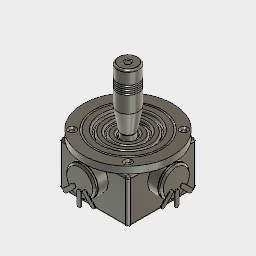
3102 Mini Joystick (Autodesk Fusion 360 design; units mm, degrees)
Autodesk Fusion 360 part; units mm, degrees
note: some values were not read from the file. Chosen so that the rebuilt part matches the saved one: which face or edge a step refers to. Set by a fixed rule: which sketch regions a step uses.
sketch "base" plane through (0, 0, 0) normal (0, 0, 1) x (1, 0, 0)
  circle A0 centre (0, 0) radius 19.8
  line L0 (16.25, -16.25) -> (-16.25, -16.25) construction
  line L1 (-16.25, -16.25) -> (-16.25, 16.25) construction
  line L2 (-16.25, 16.25) -> (16.25, 16.25) construction
  line L3 (16.25, 16.25) -> (16.25, -16.25) construction
  line L4 (16.25, -16.25) -> (-16.25, 16.25) construction
  line L5 (-16.25, -16.25) -> (16.25, 16.25) construction
  circle A1 centre (-16.25, 16.25) radius 1.25
  circle A2 centre (16.25, 16.25) radius 1.25
  circle A3 centre (16.25, -16.25) radius 1.25
  circle A4 centre (-16.25, -16.25) radius 1.25
  circle A5 centre (0, 0) radius 26
  dimension "d1" = 39.6
  dimension "d7" = 32.5
  dimension "d8" = 32.5
  dimension "d9" = 2.5
  dimension "d10" = 2.5
  dimension "d11" = 2.5
  dimension "d12" = 2.5
  dimension "d13" = 52
  measures "d1" diameter of A0
  measures "d7" distance of L1.end L2.end
  measures "d8" distance of L0.end L1.end
  measures "d9" diameter of A1
  measures "d10" diameter of A2
  measures "d11" diameter of A3
  measures "d12" diameter of A4
  measures "d13" diameter of A5
extrude "Extrude1" add sketch "base" along normal blind 4 makes body 1
sketch "stick" plane through (0, 0, 4) normal (0, 0, 1) x (-1, 0, 0)
  circle A0 centre (0, 0) radius 19.8
  circle A1 centre (0, 0) radius 4
  circle A2 centre (16.25, 16.25) radius 1.25
  circle A3 centre (16.25, -16.25) radius 1.25
  circle A4 centre (-16.25, -16.25) radius 1.25
  circle A5 centre (-16.25, 16.25) radius 1.25
  circle A6 centre (0, 0) radius 26
  dimension "d4" = 8
  measures "d4" diameter of A1
extrude "Extrude2" add sketch "stick" along normal blind 12 draft 10 separate body contours A1 makes body 2
sketch "rod" plane through (0, 0, 16) normal (0, 0, 1) x (-1, 0, 0)
  circle A0 centre (0, 0) radius 6.1159
extrude "Extrude3" add sketch "rod" along normal blind 22 bodies 2
sketch "pad (1)" plane through (0, 0, 0) normal (0, 0, 1) x (1, 0, 0)
  circle A0 centre (0, 0) radius 26
  circle A1 centre (0, 0) radius 4
  circle A2 centre (0, 0) radius 26
  circle A3 centre (0, 0) radius 19.8
  circle A4 centre (0, 0) radius 16
  circle A5 centre (0, 0) radius 12
  circle A6 centre (0, 0) radius 8
  dimension "d16" = 10
  dimension "d17" = 14
  dimension "d18" = 18
  dimension "d50" = 8
  dimension "d104" = 39.6
  measures "d50" diameter of A1
  measures "d104" diameter of A3
extrude "pad" add sketch "pad (1)" along normal blind 3 separate body contours A3 | A4 | A5 | A6 makes body 3
pipe "Pipe6" cut diameter 2 path "pad (1)" along A6 bodies 3
pipe "Pipe7" cut diameter 2 path "pad (1)" along A5 bodies 3
pipe "Pipe8" cut diameter 2 path "pad (1)" along A4 bodies 3
move_body "Move1" bodies 3 to x (-1, 0, 0) y (0, 1, 0) z (0, 0, -1) at (0, 0, 3)
ref_plane "WorkPlane1" through (0, 0, 26) normal (0, 0, 1) x (-1, 0, 0)
sketch "rings" plane through (0, 0, 26) normal (0, 0, 1) x (1, 0, 0)
  circle A0 centre (0, 0) radius 6.1159
pipe "Pipe5" cut diameter 1 path "rings" along A0 bodies 2
pattern_linear "R-Pattern1" count 3 spacing 2 along (0, 0, 1) of 1 faces at (-6.0834, 0.3036, 26.4994) on bodies 2
fillet "Fillet1" radius 1 1 edges at (5.702, 2.2116, 38) on bodies 2
extrude "Extrude5" add sketch "pad (1)" along normal blind 4 draft -10 separate body contours A1 makes body 4
fillet "Fillet2" radius 1 1 edges at (-3.0717, 1.1914, 4) on bodies 4
chamfer "Chamfer1" distance 1 angle 45 4 edges at (-17.4154, 16.702, 4) (15.0846, 16.702, 4) (-17.4154, -15.798, 4) (15.0846, -15.798, 4) on bodies 1
sketch "Sketch6" plane through (0, 0, 0) normal (0, 0, 1) x (1, 0, 0)
  line L0 (20, -20) -> (-20, -20)
  line L1 (-20, -20) -> (-20, 20)
  line L2 (-20, 20) -> (20, 20)
  line L3 (20, 20) -> (20, -20)
  line L4 (20, -20) -> (-20, 20) construction
  line L5 (-20, -20) -> (20, 20) construction
  dimension "d74" = 40
  dimension "d75" = 40
  measures "d74" distance of L1.end L2.end
  measures "d75" distance of L0.end L1.end
extrude "Extrude15" add sketch "Sketch6" against normal blind 26 separate body makes body 5
fillet "Fillet4" radius 1.5 12 edges at (20, 20, -13) (-20, 0, 0) (0, -20, -26) (20, 0, -26) (20, 0, 0) (0, 20, -26) (-20, 20, -13) (0, 20, 0) (-20, -20, -13) (0, -20, 0) (20, -20, -13) (-20, 0, -26) on bodies 5
sketch "pot a" plane through (20, 0, 0) normal (1, 0, 0) x (0, 1, 0)
  line L0 (-18.5, -1.5) -> (-18.5, -24.5)
  line L1 (-18.5, -24.5) -> (18.5, -24.5)
  line L2 (18.5, -24.5) -> (18.5, -1.5)
  line L3 (18.5, -1.5) -> (-18.5, -1.5)
  line L4 (0, -24.5) -> (0, -1.5) construction
  circle A0 centre (0, -8.5) radius 8.5
  dimension "d81" = 17
  dimension "d89" = 16
  measures "d81" diameter of A0
  measures "d89" distance of L1 A0.centre
extrude "Extrude16" add sketch "pot a" along normal blind 6 separate body contours L3 A0 | L3 A0 makes body 6
sketch "pot b" plane through (0, -20, 0) normal (0, -1, 0) x (1, 0, 0)
  line L0 (18.5, -1.5) -> (-18.5, -1.5)
  line L1 (-18.5, -1.5) -> (-18.5, -24.5)
  line L2 (-18.5, -24.5) -> (18.5, -24.5)
  line L3 (18.5, -24.5) -> (18.5, -1.5)
  line L4 (0, -1.5) -> (0, -24.5) construction
  circle A0 centre (0, -8.5) radius 8.5
  dimension "d85" = 17
  dimension "d86" = 16
  measures "d85" diameter of A0
  measures "d86" distance of L2 A0.centre
extrude "Extrude17" add sketch "pot b" along normal blind 6 separate body contours L0 A0 | L0 A0 makes body 7
fillet "Fillet5" radius 1 1 edges at (3.7293, 1.4465, 3) on bodies 3
sketch "bottom hole" plane through (0, 0, -26) normal (0, 0, -1) x (1, 0, 0)
  line L0 (18.5, -18.5) -> (18.5, 18.5)
  line L1 (18.5, 18.5) -> (-18.5, 18.5)
  line L2 (-18.5, 18.5) -> (-18.5, -18.5)
  line L3 (-18.5, -18.5) -> (18.5, -18.5)
  circle A0 centre (0, 0) radius 9.5
  dimension "d106" = 19
  measures "d106" diameter of A0
extrude "Extrude18" cut sketch "bottom hole" against normal blind 2 contours A0 bodies 5
sketch "top dimple" plane through (0, 0, 38) normal (0, 0, 1) x (-1, 0, 0)
  circle A0 centre (0, 0) radius 5.1159
  circle A1 centre (0, 0) radius 1.5
  dimension "d109" = 3
  measures "d109" diameter of A1
extrude "Extrude19" cut sketch "top dimple" against normal blind 0.5 contours A1 bodies 2
fillet "Fillet6" radius 0.5 1 edges at (1.3985, -0.5424, 38) on bodies 2
extrude "Extrude20" add sketch "pot b" along normal blind 2 from surface at 6 separate body contours L0 A0 | L0 A0 makes body 8
extrude "Extrude21" add sketch "pot a" along normal blind 2 from surface at 6 separate body contours L3 A0 | L3 A0 makes body 9
chamfer "Chamfer3" distance 1 angle 45 2 edges at (-7.9248, -28, -11.5737) (28, -7.9248, -11.5737) on bodies 8 9
chamfer "Chamfer4" distance 0.25 angle 45 2 edges at (26, -7.9248, -11.5737) (-7.9248, -26, -11.5737) on bodies 6 7
sketch "Sketch12" plane through (0, -28, 0) normal (0, -1, 0) x (1, 0, 0)
  circle A0 centre (0, -8.5) radius 7.5
  circle A1 centre (0, -8.5) radius 2
  line L0 (-1.2, -13.2) -> (-1.2, -19.8)
  arc A2 (-1.2, -19.8) -> (1.2, -19.8) centre (0, -19.8) ccw
  line L1 (1.2, -19.8) -> (1.2, -13.2)
  arc A3 (1.2, -13.2) -> (-1.2, -13.2) centre (0, -13.2) ccw
  line L2 (0, -12) -> (0, -21) construction
  line L3 (2.4749, -12.6719) -> (7.1418, -17.3388)
  arc A4 (7.1418, -17.3388) -> (8.8388, -15.6418) centre (7.9903, -16.4903) ccw
  arc A5 (4.1719, -10.9749) -> (2.4749, -12.6719) centre (3.3234, -11.8234) ccw
  line L4 (8.8388, -15.6418) -> (4.1719, -10.9749)
  line L5 (-8.8388, -15.6418) -> (-4.1719, -10.9749)
  arc A6 (-2.4749, -12.6719) -> (-4.1719, -10.9749) centre (-3.3234, -11.8234) ccw
  line L6 (-2.4749, -12.6719) -> (-7.1418, -17.3388)
  arc A7 (-8.8388, -15.6418) -> (-7.1418, -17.3388) centre (-7.9903, -16.4903) ccw
  dimension "d121" = 4
  dimension "d122" = 2.4
  dimension "d124" = 45
  measures "d121" diameter of A1
  measures "d122" diameter of A2
extrude "Extrude22" add sketch "Sketch12" along normal blind 0.5 separate body contours A0 L5 A6 L6 | A0 L5 L6 A7 | A0 L3 A4 L4 | A0 L3 A5 L4 | A0 L0 L1 A3 | A0 L0 A2 L1 makes body 10 at (-4.5962, -28, -13.6619) makes body 11 at (0.4, -28, -15.4) makes body 12 at (4.5962, -28.5, -13.6619)
sketch "Sketch13" plane through (28, 0, 0) normal (1, 0, 0) x (0, 1, 0)
  circle A0 centre (0, -8.5) radius 7.5
  circle A1 centre (0, -8.5) radius 2
  line L0 (-1.2, -13.2) -> (-1.2, -19.8)
  arc A2 (-1.2, -19.8) -> (1.2, -19.8) centre (0, -19.8) ccw
  line L1 (1.2, -19.8) -> (1.2, -13.2)
  arc A3 (1.2, -13.2) -> (-1.2, -13.2) centre (0, -13.2) ccw
  line L2 (0, -12) -> (0, -21) construction
  line L3 (2.4749, -12.6719) -> (7.1418, -17.3388)
  arc A4 (7.1418, -17.3388) -> (8.8388, -15.6418) centre (7.9903, -16.4903) ccw
  line L4 (8.8388, -15.6418) -> (4.1719, -10.9749)
  arc A5 (4.1719, -10.9749) -> (2.4749, -12.6719) centre (3.3234, -11.8234) ccw
  line L5 (-8.8388, -15.6418) -> (-4.1719, -10.9749)
  arc A6 (-2.4749, -12.6719) -> (-4.1719, -10.9749) centre (-3.3234, -11.8234) ccw
  arc A7 (-8.8388, -15.6418) -> (-7.1418, -17.3388) centre (-7.9903, -16.4903) ccw
  line L6 (-2.4749, -12.6719) -> (-7.1418, -17.3388)
  dimension "d127" = 4
  dimension "d128" = 2.4
  dimension "d130" = 45
  measures "d127" diameter of A1
  measures "d128" diameter of A2
extrude "Extrude23" add sketch "Sketch13" along normal blind 0.5 separate body contours A0 L5 A6 L6 | A0 L5 A7 L6 | A0 L3 A4 L4 | A0 L3 L4 A5 | A0 L0 L1 A3 | A0 L0 A2 L1 makes body 13 at (28, -4.5962, -13.6619) makes body 14 at (28, 0.4, -17.6) makes body 15 at (28, 4.5962, -13.6619)
sketch "Sketch15" plane through (0, 0, 0) normal (1, 0, 0) x (0, 1, 0)
  line L0 (19.8, 4) -> (14.8, 4)
  line L1 (14.8, 4) -> (14.8, 3)
  line L2 (14.8, 3) -> (9.8, 3)
  line L3 (9.8, 3) -> (9.8, 2)
  line L4 (9.8, 2) -> (4.8, 2)
  line L5 (4.8, 2) -> (4.8, 1)
  line L6 (4.8, 1) -> (0, 1)
  line L7 (0, 1) -> (0, 0)
  line L8 (19.8, 0) -> (19.8, 4)
  line L9 (0, 0) -> (19.8, 0)
  line L10 (14.8, 3) -> (13.8, 3)
  line L11 (13.8, 3) -> (13.8, 0)
  line L12 (13.8, 0) -> (14.8, 0)
  line L13 (14.8, 0) -> (14.8, 3)
  line L14 (9.8, 2) -> (8.8, 2)
  line L15 (8.8, 2) -> (8.8, 0)
  line L16 (8.8, 0) -> (9.8, 0)
  line L17 (9.8, 0) -> (9.8, 2)
  line L18 (4.8, 1) -> (3.8, 1)
  line L19 (3.8, 1) -> (3.8, 0)
  line L20 (3.8, 0) -> (4.8, 0)
  line L21 (4.8, 0) -> (4.8, 1)
  line L22 (19.8, 4) -> (18.8, 4)
  line L23 (18.8, 4) -> (18.8, 0)
  line L24 (18.8, 0) -> (19.8, 0)
  line L25 (19.8, 0) -> (19.8, 4)
  dimension "d134" = 5
  dimension "d135" = 4
  dimension "d136" = 1
  dimension "d137" = 1
  dimension "d138" = 1
  dimension "d139" = 19.8
  dimension "d141" = 5
  dimension "d142" = 5
  dimension "d143" = 1
  dimension "d144" = 1
  dimension "d145" = 1
  dimension "d150" = 1
  measures "d134" distance of L0.start L0.end
  measures "d135" distance of L0.start L8.start
  measures "d136" distance of L0.end L1.end
  measures "d137" distance of L2.end L3.end
  measures "d138" distance of L4.end L5.end
  measures "d139" distance of L7.end L8.start
  measures "d141" distance of L1.end L2.end
  measures "d142" distance of L3.end L4.end
  measures "d143" distance of L1.end L10.end
  measures "d144" distance of L3.end L14.end
  measures "d145" distance of L5.end L18.end
  measures "d150" distance of L0.start L22.end
revolve "Revolve1" add sketch "Sketch15" angle 360 about axis through (0, 0, 1.75) along (0, 0, 1) separate body contours L0 L8 L9 L22 L23 L24 L25 | L0 L1 L9 L13 L23 | L2 L3 L9 L11 L17 | L4 L5 L9 L15 L21 | L6 L7 L9 L19 makes body 16 at (0.6856, 12.4153, 0) makes body 17 at (0.4372, 7.4339, 0) makes body 18 at (0.9837, 18.0596, 0) makes body 19 at (-1.0687, -0.4461, 0)
extrude "Extrude24" add sketch "pad (1)" along normal blind 0.5 contours A1 | A3 | A4 | A5 | A6 bodies 16 17 18 19
fillet "Fillet7" radius 1 7 edges at (-13.7984, 5.3519, 4) (-12.8661, 4.9903, 3) (-9.1368, 3.5438, 3) (-8.2045, 3.1822, 2) (-4.4752, 1.7358, 2) (-3.5428, 1.3741, 1) (-18.4601, 7.16, 4) on bodies 16 17 18 19
delete_body "RemoveBody1" bodies 3
fillet "Fillet8" radius 0.5 5 edges at (5.3519, -13.7984, 0.5) (4.9903, -12.8661, 0.5) (-3.1822, -8.2045, 0.5) (-3.5438, -9.1368, 0.5) (1.7358, -4.4752, 0.5) on bodies 16
equation "d8 = d7"
equation "d9 = holes"
equation "d10 = holes"
equation "d11 = holes"
equation "d12 = holes"
equation "d74 = box"
equation "d75 = box"
equation "holes = 2.5 mm"
equation "box = 40 mm"
equation "d81 = pots"
equation "d85 = pots"
equation "pots = 17 mm"
equation "ring = 53 mm"
equation "d137 = d136"
equation "d138 = d136"
named bodies: "base", "stick", "pad", "nub", "box", "pot a", "pot b", "cap a", "cap b"
